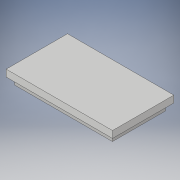
# Autodesk Inventor part: Cap
Saved by Autodesk Inventor 2019 (Build 230136000, 136)
## iProperties
Created: 2019-04-15
Part Number: Cap
Material: Generic
Document SubType Name: Modeling
Designer: Epsilon
Density: 1 g/cm^3
Appearance: Default
Author: Epsilon
Autodesk Inventor part; units mm, degrees
ref_plane "YZ Plane" through (0, 0, 0) normal (1, 0, 0) x (0, 1, 0)
ref_plane "XZ Plane" through (0, 0, 0) normal (0, 1, 0) x (-1, 0, 0)
ref_plane "XY Plane" through (0, 0, 0) normal (0, 0, 1) x (1, 0, 0)
sketch "Sketch1" plane through (0, 0, 0) normal (0, 1, 0) x (-1, 0, 0)
  line L0 (0, 0) -> (72, 0)
  line L1 (72, 0) -> (72, -39)
  line L2 (72, -39) -> (0, -39)
  line L3 (0, -39) -> (0, 0)
  dimension "d0" = 72
  dimension "d1" = 39
  constraints: 8 end point, 2 parallel, 1 horizontal, 1 perpendicular
  measures "d0" distance of L1.end L2.end
  measures "d1" distance between parallel lines of L2 L0
extrude "Extrusion1" add sketch "Sketch1" along normal blind 5
sketch "Sketch2" plane through (0, 5, 0) normal (0, 1, 0) x (1, 0, 0)
  line L0 (-75, -3) -> (3, -3)
  line L1 (3, -3) -> (3, 42)
  line L2 (3, 42) -> (-75, 42)
  line L3 (-75, 42) -> (-75, -3)
  line L4 (-72, 0) -> (0, 0) projected
  line L5 (-72, 39) -> (-72, 0) projected
  line L6 (0, 39) -> (-72, 39) projected
  line L7 (0, 0) -> (0, 39) projected
  dimension "d4" = 3
  dimension "d5" = 3
  dimension "d6" = 3
  dimension "d7" = 3
  constraints: 8 end point, 2 parallel, 1 horizontal, 1 perpendicular
  measures "d4" distance between parallel lines of L0 L4
  measures "d5" distance between parallel lines of L5 L3
  measures "d6" distance between parallel lines of L2 L6
  measures "d7" distance between parallel lines of L1 L7
extrude "Extrusion2" add sketch "Sketch2" along normal blind 5 contours L3 L2 L1 L0 | L5 L6 L7 L4
equation "\"d5\" = d4"
equation "\"d6\" = d4"
equation "\"d7\" = d4"
body "Solid1"
